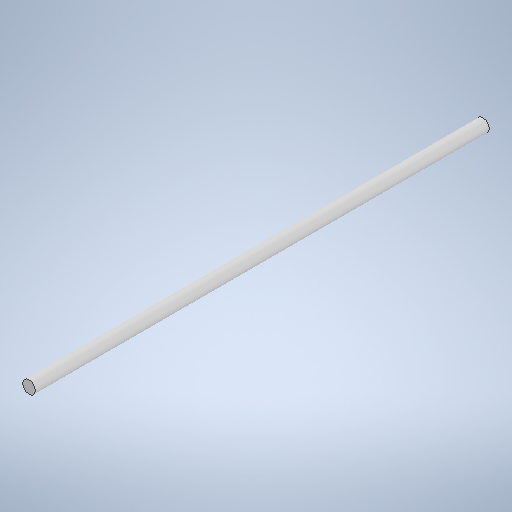
# Autodesk Inventor part: szpilka
Saved by Autodesk Inventor 2025.2 (Build 292293000, 293)
## iProperties
Created: 2025-11-26
Part Number: szpilka
Material: Ogólny
Document SubType Name: Modeling
Designer: juras
Density: 1 g/cm^3
Appearance: Domyślna
Author: juras
Autodesk Inventor part; units mm, degrees
ref_plane "YZ Plane" through (0, 0, 0) normal (1, 0, 0) x (0, 1, 0)
ref_plane "XZ Plane" through (0, 0, 0) normal (0, 1, 0) x (-1, 0, 0)
ref_plane "XY Plane" through (0, 0, 0) normal (0, 0, 1) x (1, 0, 0)
sketch "Szkic2" plane through (0, 0, 0) normal (0, 1, 0) x (-1, 0, 0)
  line L0 (0, 0) -> (0, 250)
  line L1 (0, 250) -> (-3.5, 250)
  line L2 (-3.5, 250) -> (-3.5, 0)
  line L3 (-3.5, 0) -> (0, 0)
  line L4 (0, 0) -> (0, 0)
  dimension "d4" = 250
  dimension "d5" = 3.5
  dimension "d6" = 250
  dimension "d7" = 90
  dimension "d8" = 3.5
  constraints: 10 end point, 1 horizontal, 1 parallel, 1 perpendicular, 1 vertical
  measures "d4" distance of L0.start L0.end
  measures "d5" distance of L0.end L1.end
  measures "d6" distance of L1.end L2.end
  measures "d7" angle of L2 L1
  measures "d8" distance of L2.end L3.end
revolve "Obrót1" add sketch "Szkic2" angle 360 about axis through (0, 0, 0) along (0, 0, 1)
